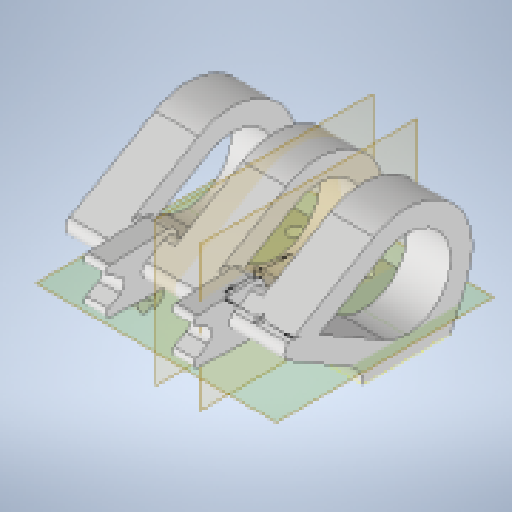
# Autodesk Inventor part: PenHolder
Saved by Autodesk Inventor 2023 (Build 270158000, 158)
## iProperties
Created: 2023-09-03
Part Number: PenHolder
Material: Generic
Document SubType Name: Modeling
Designer: Felix
Density: 1 g/cm^3
Appearance: Default
Author: Felix
Autodesk Inventor part; units mm, degrees
ref_plane "YZ Plane" through (0, 0, 0) normal (1, 0, 0) x (0, 1, 0)
ref_plane "XZ Plane" through (0, 0, 0) normal (0, 1, 0) x (-1, 0, 0)
ref_plane "XY Plane" through (0, 0, 0) normal (0, 0, 1) x (1, 0, 0)
sketch "Sketch3" plane through (0, 0, 0) normal (1, 0, 0) x (0, 1, 0)
  line L0 (6.3397, 0) -> (23.6603, 0) construction
  line L1 (23.6603, 0) -> (15, 15)
  line L2 (15, 15) -> (6.3397, 0)
  arc A0 (6.3397, 0) -> (23.6603, 0) centre (15, -5) ccw
  line L3 (0, -15) -> (0, 5)
  line L4 (5.1795, 7.9904) -> (15, 25)
  line L5 (15, 25) -> (27.9904, 2.5)
  arc A1 (9.2308, -18.8462) -> (27.9904, 2.5) centre (15, -5) ccw
  line L6 (0, -15) -> (9.2308, -18.8462)
  arc A2 (0, 5) -> (5.1795, 7.9904) centre (0, 10.9808) ccw
  point P0 (0, 0)
  point P1 (0, 0)
  point P2 (15, 0)
  point P3 (0, -5)
  dimension "d18" = 60
  dimension "d19" = 10
  dimension "d20" = 20
  dimension "d21" = 5
  dimension "d22" = 5
  dimension "d23" = 5
  constraints: 14 end point, 6 point on circle, 4 tangent, 3 centre point, 3 midpoint, 2 horizontal alignment, 2 parallel, 2 vertical alignment, 1 coincident, 1 horizontal, 1 line through centre, 1 vertical
  measures "d18" angle of L2 L1
  measures "d19" radius of A0
  measures "d20" distance of L3.start L3.end
  measures "d21" distance edge to line of A0 L3
  measures "d22" radial gap between concentric circles of A1 A0
  measures "d23" distance between parallel lines of L2 L4
extrude "Extrusion3" add sketch "Sketch3" along normal blind 50
ref_plane "Work Plane2" through (0, 5, -5) normal (0, -1, 0) x (1, 0, 0)
sketch "Sketch4" plane through (0, 5, -5) normal (0, -1, 0) x (1, 0, 0)
  line L0 (0, 30) -> (50, 30) construction
  line L1 (50, 7.5) -> (50, 30) construction
  line L2 (50, 30) -> (50, 12.9904) construction
  line L3 (50, 12.9904) -> (50, 10) construction
  line L4 (50, 10) -> (50, -10) construction
  line L5 (50, -10) -> (50, -13.8462) construction
  line L6 (50, -13.8462) -> (50, 7.5) construction
  line L7 (50, 5) -> (50, 5) construction
  line L8 (50, 5) -> (50, 20) construction
  line L9 (50, 20) -> (50, 5) construction
  line L10 (0, 7.5) -> (0, 30) construction
  line L11 (0, -13.8462) -> (0, 7.5) construction
  line L12 (0, -10) -> (0, -13.8462) construction
  line L13 (0, 10) -> (0, -10) construction
  line L14 (0, 12.9904) -> (0, 10) construction
  line L15 (0, 30) -> (0, 12.9904) construction
  line L16 (0, 5) -> (0, 5) construction
  line L17 (0, 20) -> (0, 5) construction
  line L18 (0, 5) -> (0, 20) construction
  line L19 (40, -20) -> (30, -20)
  line L20 (30, -20) -> (30, 20)
  line L21 (30, 20) -> (40, 20)
  line L22 (40, 20) -> (40, -20)
  line L23 (20, -20) -> (10, -20)
  line L24 (10, -20) -> (10, 20)
  line L25 (10, 20) -> (20, 20)
  line L26 (20, 20) -> (20, -20)
  line L27 (0, 20) -> (0, 5) construction
  line L28 (0, 5) -> (50, 5) construction
  line L29 (50, 20) -> (50, 5) construction
  line L30 (0, 20) -> (50, 20) construction
  line L31 (25, -13.8462) -> (25, 30) construction
  dimension "d26" = 10
  dimension "d27" = 10
  dimension "d28" = 10
  dimension "d29" = 10
  dimension "d32" = 40
  constraints: 18 end point, 4 parallel, 2 horizontal, 2 perpendicular, 2 point on line, 1 collinear, 1 midpoint, 1 other
  measures "d26" distance between parallel lines of L24 L26
  measures "d27" distance between parallel lines of L20 L22
  measures "d28" distance between parallel lines of L26 L20
  measures "d29" distance between parallel lines of L11 L24
  measures "d32" distance between parallel lines of L30 L19
extrude "Extrusion4" cut sketch "Sketch4" against normal blind 50
ref_plane "Work Plane3" through (35, 20.7735, 15) normal (1, 0, 0) x (0, 0, -1)
ref_plane "Work Plane4" through (25, 15, 25) normal (1, 0, 0) x (0, 0, -1)
sketch "Sketch5" plane through (35, 20.7735, 15) normal (1, 0, 0) x (0, 0, -1)
  line L0 (12.5, 7.2169) -> (-10, -5.7735) projected
  line L1 (-10, -5.7735) -> (7.0096, -15.594) construction
  arc A0 (10, -20.7735) -> (7.0096, -15.594) centre (4.0192, -20.7735) ccw construction
  line L2 (10, -20.7735) -> (30, -20.7735) construction
  line L3 (30, -20.7735) -> (33.8462, -11.5427) construction
  arc A1 (33.8462, -11.5427) -> (12.5, 7.2169) centre (20, -5.7735) ccw construction
  arc A2 (15, -14.4338) -> (15, 2.8868) centre (20, -5.7735) ccw construction
  line L4 (15, -14.4338) -> (0, -5.7735) construction
  line L5 (0, -5.7735) -> (15, 2.8868) construction
  line L6 (-10, -5.7735) -> (-15.6768, -2.496)
  line L7 (12.5, 7.2169) -> (0, 0) projected
  line L8 (0, -11.547) -> (7.0096, -15.594) projected
  line L9 (0, 0) -> (0, -11.547) construction
  line L10 (-15.2182, -0.6308) -> (0, 0)
  line L11 (0, -5.7735) -> (15, -14.4338) projected
  line L12 (0, -5.7735) -> (-10, -5.7735) construction
  line L13 (-10, -5.7735) -> (0, 0)
  line L14 (-10, -5.7735) -> (-15.6768, -9.051)
  line L15 (-15.2182, -10.9162) -> (0, -11.547)
  line L16 (-10, -5.7735) -> (0, -11.547)
  arc A3 (-15.2182, -0.6308) -> (-15.6768, -2.496) centre (-15.1768, -1.63) ccw
  arc A4 (-15.6768, -9.051) -> (-15.2182, -10.9162) centre (-15.1768, -9.917) ccw
  point P0 (15, -20.7735)
  point P1 (-18.6603, -0.7735)
  point P2 (-18.6603, -10.7735)
  dimension "d33" = 180
  dimension "d34" = 10
  dimension "d37" = 1
  constraints: 16 end point, 4 point on circle, 4 point on line, 4 tangent, 2 centre point, 1 collinear, 1 equal radius, 1 horizontal, 1 symmetric about line
  measures "d33" angle of L6 L1
  measures "d34" distance of point (-18.66, -10.774) point (-18.66, -0.774)
  measures "d37" radius of A3
extrude "Extrusion5" add sketch "Sketch5" along normal mid plane 5
fillet "Fillet3" radius 2 7 edges at (38.75, 9.2265, 15) (31.25, 9.2265, 15) (35, 9.2265, 15) (38.75, 20.7735, 15) (31.25, 20.7735, 15) (35, 20.7735, 15) (35, 15, 25)
mirror "Mirror2" about plane through (25, 15, 25) normal (1, 0, 0) of "Extrusion5"
fillet "Fillet5" radius 2 7 edges at (15, 15, 25) (11.25, 20.7735, 15) (18.75, 20.7735, 15) (15, 20.7735, 15) (11.25, 9.2265, 15) (18.75, 9.2265, 15) (15, 9.2265, 15)
fillet "Fillet4" radius 2 3 edges at (43.75, 15, 25) (25, 15, 25) (6.25, 15, 25)
sketch "Sketch6" plane through (0, 0, -15) normal (0, -1, 0) x (1, 0, 0)
  line L0 (0, 20) -> (0, 0) construction
  line L1 (0, 0) -> (50, 0) construction
  line L2 (50, 20) -> (50, 0) construction
  line L3 (0, 20) -> (50, 20) construction
  line L4 (50, 20) -> (0, 0) construction
  line L5 (0, 20) -> (50, 0) construction
  line L6 (33, 2.5) -> (17, 2.5) construction
  line L7 (17, 2.5) -> (17, 17.5) construction
  line L8 (17, 17.5) -> (33, 17.5) construction
  line L9 (33, 17.5) -> (33, 2.5) construction
  line L10 (33, 2.5) -> (17, 17.5) construction
  line L11 (17, 2.5) -> (33, 17.5) construction
  point P0 (0, 15)
  point P1 (25, 10)
  dimension "d43" = 16
  dimension "d44" = 15
  constraints: 16 end point, 3 midpoint, 2 parallel, 1 horizontal, 1 perpendicular
  measures "d43" distance of L7.end L8.end
  measures "d44" distance of L6.end L7.end
sketch "Sketch7" plane through (0, 5, -5) normal (0, 1, 0) x (1, 0, 0)
  point P0 (0, -5)
  point P1 (33, -7.5)
  point P2 (17, -7.5)
  point P3 (17, 7.5)
  point P4 (33, 7.5)
hole "Hole1" at (17, 5, -12.5) at (17, 5, 2.5) at (33, 5, 2.5) at (33, 5, -12.5) direction (0, -1, 0) diameter 3.2 depth 8 clearance for "Countersunk Flat Head Screw DIN EN ISO 2009" size "M3" standard "DIN"
sketch "Sketch9" plane through (0, 0, 0) normal (-1, 0, 0) x (0, 0, 1)
  line L0 (5, 0) -> (-15, 0) projected
  arc A0 (7.9904, 5.1795) -> (5, 0) centre (10.9808, 0) ccw projected
  line L1 (22, 13.2679) -> (7.9904, 5.1795) projected
  arc A1 (7.3612, -10.25) -> (7.3612, -1.75) centre (0, -6) ccw construction
  line L2 (6, -6) -> (11, -6)
  line L3 (5, 0) -> (-15, 0) projected
  line L4 (6, -6) -> (5, 0)
  line L5 (11, -6) -> (12.9952, 8.069)
  line L6 (18, 10.9585) -> (7.9904, 5.1795) projected
  circle A2 centre (8.5, -3) radius 1
  circle A3 centre (8.5, -6) radius 0.75
  arc A4 (7.3612, -10.25) -> (7.3612, -1.75) centre (0, -6) ccw
  point P0 (0, 0)
  point P1 (7.75, -6)
  point P2 (9.25, -6)
  dimension "d55" = 5
  dimension "d56" = 2
  dimension "d57" = 2
  dimension "d61" = 1.5
  constraints: 6 end point, 5 point on circle, 4 centre point, 4 midpoint, 2 coincident, 1 concentric, 1 horizontal, 1 horizontal alignment, 1 vertical alignment, 4 other
  measures "d55" distance of L2.start L2.end
  measures "d56" diameter of A2
  measures "d57" distance edge to line of A2 L2
  measures "d61" diameter of A3
extrude "Extrusion7" add sketch "Sketch9" against normal blind 5 contours L1 L5 L2 A3 L4 A0
fillet "Fillet6" radius 2 3 edges at (2.5, -6, 11) (2.5, 8.069, 12.9952) (2.5, -6, 6)
equation "\"d23\" = d22"
equation "\"d27\" = d26"
equation "\"d28\" = d29"
body "Solid3"
